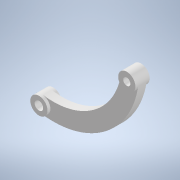
# Autodesk Inventor part: Part4
Saved by Autodesk Inventor 2020 (Build 240168000, 168)
## iProperties
Created: 2019-08-12
Part Number: Part4
Material: Generic
Document SubType Name: Modeling
Designer: Horváth Patrik
Density: 1 g/cm^3
Appearance: Default
Author: Horváth Patrik
Autodesk Inventor part; units mm, degrees
ref_plane "YZ Plane" through (0, 0, 0) normal (1, 0, 0) x (0, 1, 0)
ref_plane "XZ Plane" through (0, 0, 0) normal (0, 1, 0) x (-1, 0, 0)
ref_plane "XY Plane" through (0, 0, 0) normal (0, 0, 1) x (1, 0, 0)
sketch "Sketch1" plane through (0, 0, 0) normal (0, 0, 1) x (1, 0, 0)
  circle A0 centre (36.1927, 22.6099) radius 1.25 projected
  circle A1 centre (36.1927, 22.6099) radius 3
  circle A2 centre (5.9801, 40.2425) radius 1.4795 projected
  circle A3 centre (5.9801, 40.2425) radius 3
  point P0 (0, 0)
  dimension "d9" = 6
  constraints: 2 centre point, 2 coincident, 1 equal radius
  measures "d9" diameter of A3
extrude "Extrusion1" add sketch "Sketch1" along normal blind 1
sketch "Sketch5" plane through (5.9801, 40.2425, 1) normal (0, 0, 1) x (1, 0, 0)
  circle A0 centre (0, 0) radius 3 projected
  circle A1 centre (0, 0) radius 1.4795 projected
  circle A2 centre (30.2126, -17.6326) radius 3 projected
  circle A3 centre (30.2126, -17.6326) radius 1.25 projected
  arc A4 (0, 0) -> (30.2126, -17.6326) centre (29.2115, 15.3522) ccw construction
  arc A5 (-2.6556, -1.3957) -> (30.3036, -20.6312) centre (29.2115, 15.3522) ccw
  arc A6 (2.6556, 1.3957) -> (30.1216, -14.634) centre (29.2115, 15.3522) ccw
  arc A7 (2.6556, 1.3957) -> (-2.6556, -1.3957) centre (0, 0) ccw
  arc A8 (30.3036, -20.6312) -> (30.1216, -14.634) centre (30.2126, -17.6326) ccw
  circle A9 centre (30.2126, -17.6326) radius 3 projected
  point P0 (-5.9801, -40.2425)
  point P1 (30.1216, -14.634)
  point P2 (2.6556, 1.3957)
  point P3 (-2.6556, -1.3957)
  point P4 (30.3036, -20.6312)
  dimension "d10" = 30
  constraints: 10 point on circle, 5 centre point, 4 tangent, 1 concentric
  measures "d10" radius of A6
extrude "Extrusion4" add sketch "Sketch5" along normal blind 3
body "Solid1"
